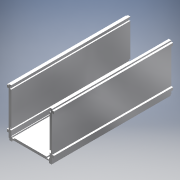
# Autodesk Inventor part: CompactSlidePart2
Saved by Autodesk Inventor 2019 (Build 230136000, 136)
## iProperties
Created: 2017-11-11
Part Number: CompactSlidePart2
Material: Aluminum 6061
Document SubType Name: Modeling
Designer: User
Density: 2.7 g/cm^3
Appearance: Aluminum - Flat
Mass: 1808.92 g
Surface Area: 2425.07 cm^2
Volume: 669.969 cm^3
Author: User
Autodesk Inventor part; units mm, degrees
ref_plane "YZ Plane" through (0, 0, 0) normal (1, 0, 0) x (0, 1, 0)
ref_plane "XZ Plane" through (0, 0, 0) normal (0, 1, 0) x (-1, 0, 0)
ref_plane "XY Plane" through (0, 0, 0) normal (0, 0, 1) x (1, 0, 0)
sketch "Sketch1" plane through (0, 0, 0) normal (0, 0, 1) x (1, 0, 0)
  line L0 (111.125, 0) -> (104.775, 0)
  line L1 (6.35, 0) -> (0, 0)
  line L2 (0, 0) -> (0, -3.175)
  line L3 (0, -3.175) -> (-4.7752, -3.175)
  line L4 (-4.7752, -3.175) -> (-4.7752, -9.525)
  line L5 (-4.7752, -9.525) -> (0, -9.525)
  line L6 (0, -119.0625) -> (0, -107.9373)
  line L7 (0, -107.9373) -> (-4.7752, -107.9373)
  line L8 (-4.7752, -107.9373) -> (-4.7752, -101.5873)
  line L9 (-4.7752, -101.5873) -> (0, -101.5873)
  line L10 (0, -119.0625) -> (1.5875, -119.0625)
  line L11 (1.5875, -119.0625) -> (1.5875, -123.8377)
  line L12 (1.5875, -123.8377) -> (7.9375, -123.8377)
  line L13 (7.9375, -123.8377) -> (7.9375, -119.0625)
  line L14 (0, 0) -> (0, -3.175)
  line L15 (0, -9.525) -> (0, -101.5873)
  line L16 (0, -107.9373) -> (0, -119.0625)
  line L17 (0, -119.0625) -> (1.5875, -119.0625)
  line L18 (111.125, -3.175) -> (115.9002, -3.175)
  line L19 (115.9002, -3.175) -> (115.9002, -9.525)
  line L20 (115.9002, -9.525) -> (111.125, -9.525)
  line L21 (111.125, -3.175) -> (111.125, 0)
  line L22 (111.125, -107.9373) -> (115.9002, -107.9373)
  line L23 (115.9002, -107.9373) -> (115.9002, -101.5873)
  line L24 (115.9002, -101.5873) -> (111.125, -101.5873)
  line L25 (111.125, -119.0625) -> (111.125, -107.9373)
  line L26 (111.125, -101.5873) -> (111.125, -9.525)
  line L27 (111.125, -119.0625) -> (109.5375, -119.0625)
  line L28 (109.5375, -119.0625) -> (109.5375, -123.8377)
  line L29 (109.5375, -123.8377) -> (103.1875, -123.8377)
  line L30 (103.1875, -123.8377) -> (103.1875, -119.0625)
  line L31 (7.9375, -119.0625) -> (103.1875, -119.0625)
  line L32 (109.5375, -119.0625) -> (111.125, -119.0625)
  line L33 (6.35, -3.175) -> (3.175, -3.175)
  line L34 (3.175, -3.175) -> (3.175, -9.525)
  line L35 (3.175, -9.525) -> (6.35, -9.525)
  line L36 (6.35, -3.175) -> (6.35, 0)
  line L37 (104.775, -3.175) -> (107.95, -3.175)
  line L38 (107.95, -3.175) -> (107.95, -9.525)
  line L39 (107.95, -9.525) -> (104.775, -9.525)
  line L40 (104.775, 0) -> (104.775, -3.175)
  line L41 (6.35, -112.7125) -> (6.35, -100.0125)
  line L42 (6.35, -100.0125) -> (3.175, -100.0125)
  line L43 (3.175, -100.0125) -> (3.175, -93.6625)
  line L44 (3.175, -93.6625) -> (6.35, -93.6625)
  line L45 (6.35, -112.7125) -> (6.35, -100.0125)
  line L46 (6.35, -93.6625) -> (6.35, -9.525)
  line L47 (6.35, -112.7125) -> (7.9375, -112.7125)
  line L48 (7.9375, -112.7125) -> (7.9375, -115.8875)
  line L49 (7.9375, -115.8875) -> (14.2875, -115.8875)
  line L50 (14.2875, -115.8875) -> (14.2875, -112.7125)
  line L51 (7.9375, -112.7125) -> (6.35, -112.7125)
  line L52 (104.775, -112.7125) -> (103.1875, -112.7125)
  line L53 (103.1875, -112.7125) -> (103.1875, -115.8875)
  line L54 (103.1875, -115.8875) -> (96.8375, -115.8875)
  line L55 (96.8375, -115.8875) -> (96.8375, -112.7125)
  line L56 (104.775, -112.7125) -> (103.1875, -112.7125)
  line L57 (96.8375, -112.7125) -> (14.2875, -112.7125)
  line L58 (104.775, -112.7125) -> (104.775, -100.0125)
  line L59 (104.775, -100.0125) -> (107.95, -100.0125)
  line L60 (107.95, -100.0125) -> (107.95, -93.6625)
  line L61 (107.95, -93.6625) -> (104.775, -93.6625)
  line L62 (104.775, -9.525) -> (104.775, -93.6625)
  line L63 (104.775, -100.0125) -> (104.775, -112.7125)
  dimension "d0" = 119.0625
  dimension "d1" = 111.125
  dimension "d2" = 6.35
  dimension "d3" = 112.7125
  dimension "d4" = 98.425
  dimension "d7" = 119.0625
  dimension "d10" = 3.175
  dimension "d11" = 4.7752
  dimension "d12" = 6.35
  dimension "d13" = 11.1252
  dimension "d14" = 4.7752
  dimension "d15" = 6.35
  dimension "d16" = 1.5875
  dimension "d17" = 4.7752
  dimension "d18" = 6.35
  dimension "d19" = 4.7752
  dimension "d20" = 4.7752
  dimension "d21" = 1.5875
  dimension "d22" = 6.35
  dimension "d24" = 3.175
  dimension "d25" = 3.175
  dimension "d26" = 12.7
  dimension "d27" = 6.35
  dimension "d28" = 1.5875
  dimension "d29" = 3.175
  dimension "d30" = 6.35
  dimension "d31" = 1.5875
  dimension "d32" = 6.35
  dimension "d33" = 12.7
  dimension "d34" = 6.35
  constraints: 128 end point, 87 perpendicular, 16 parallel, 5 horizontal, 3 vertical, 1 point on line
  measures "d0" distance of L1.end L6.start
  measures "d1" distance of L6.start L25.start
  measures "d2" distance of L0.start L0.end
  measures "d3" distance of L0.end L52.start
  measures "d4" distance of L52.start L41.start
  measures "d7" distance of L25.start L0.start
  measures "d10" distance of L1.end L2.end
  measures "d11" distance of L2.end L3.end
  measures "d12" distance of L3.end L4.end
  measures "d13" distance of L6.start L6.end
  measures "d14" distance of L6.end L7.end
  measures "d15" distance of L7.end L8.end
  measures "d16" distance of L6.start L10.end
  measures "d17" distance of L10.end L11.end
  measures "d18" distance of L11.end L12.end
  measures "d19" distance of L18.start L18.end
  measures "d20" distance of L22.start L22.end
  measures "d21" distance of L25.start L27.end
  measures "d22" distance of L28.end L29.end
  measures "d24" distance of L33.start L33.end
  measures "d25" distance of L37.start L37.end
  measures "d26" distance of L41.start L41.end
  measures "d27" distance of L42.end L43.end
  measures "d28" distance of L41.start L47.end
  measures "d29" distance of L47.end L48.end
  measures "d30" distance of L48.end L49.end
  measures "d31" distance of L52.start L52.end
  measures "d32" distance of L53.end L54.end
  measures "d33" distance of L52.start L58.end
  measures "d34" distance of L59.end L60.end
extrude "Extrusion1" add sketch "Sketch1" along normal blind 304.8
body "Solid1"
